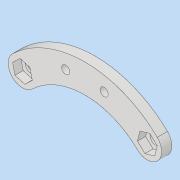
# Autodesk Inventor part: gearboxBearingHolderHexNutBacking
Saved by Autodesk Inventor 2017.3 (Build 213256000, 256)
## iProperties
Created: 2018-09-03
Part Number: gearboxBearingHolderHexNutBacking
Material: ABS Plastic
Document SubType Name: Modeling
Designer: Derek Wider
Density: 1.06 g/cm^3
Appearance: Smooth - White
Author: Derek Wider
Autodesk Inventor part; units mm, degrees
ref_plane "YZ Plane" through (0, 0, 0) normal (1, 0, 0) x (0, 1, 0)
ref_plane "XZ Plane" through (0, 0, 0) normal (0, 1, 0) x (-1, 0, 0)
ref_plane "XY Plane" through (0, 0, 0) normal (0, 0, 1) x (1, 0, 0)
sketch "Sketch1" plane through (0, 0, 0) normal (0, 0, 1) x (1, 0, 0)
  line L0 (-2.3083, -2.2118) -> (-3.0696, 0.8931)
  line L1 (-3.0696, 0.8931) -> (-0.7613, 3.1049)
  line L2 (-0.7613, 3.1049) -> (2.3083, 2.2118)
  line L3 (2.3083, 2.2118) -> (3.0696, -0.8931)
  line L4 (3.0696, -0.8931) -> (0.7613, -3.1049)
  line L5 (0.7613, -3.1049) -> (-2.3083, -2.2118)
  line L6 (41.9062, 0.8931) -> (41.1449, -2.2118)
  line L7 (41.1449, -2.2118) -> (38.0753, -3.1049)
  line L8 (38.0753, -3.1049) -> (35.767, -0.8931)
  line L9 (35.767, -0.8931) -> (36.5283, 2.2118)
  line L10 (36.5283, 2.2118) -> (39.5979, 3.1049)
  line L11 (39.5979, 3.1049) -> (41.9062, 0.8931)
  circle A0 centre (0, 0) radius 4.445
  circle A1 centre (38.8366, 0) radius 4.445
  arc A2 (41.9119, 3.2095) -> (-3.0753, 3.2095) centre (19.4183, -20.2654) ccw
  arc A3 (35.7613, -3.2095) -> (3.0753, -3.2095) centre (19.4183, -20.2654) ccw
  arc A4 (38.8366, 0) -> (0, 0) centre (19.4183, -20.2654) ccw construction
  line L12 (-1.9155, 1.999) -> (-3.0753, 3.2095) construction
  line L13 (40.7521, 1.999) -> (41.9119, 3.2095) construction
  circle A5 centre (13.4501, 7.1597) radius 1.27
  circle A6 centre (25.3865, 7.1597) radius 1.27
  dimension "d0" = 38.8366
  dimension "d1" = 5.5372
  dimension "d2" = 8.89
  dimension "d3" = 28.067
  dimension "d8" = 2.54
  dimension "d9" = 2.54
  dimension "d10" = 31.5
  dimension "d11" = 31.5
  constraints: 28 end point, 12 point on circle, 7 centre point, 5 coincident, 4 tangent, 2 line through centre, 2 midpoint, 2 perpendicular, 1 equal length, 1 equal radius, 1 horizontal alignment, 26 other
  measures "d0" distance of point (38.837, 0) point (0, 0)
  measures "d1" distance between parallel lines of L7 L10
  measures "d2" diameter of A0
  measures "d3" radius of A4
  measures "d8" diameter of A5
  measures "d9" diameter of A6
extrude "Extrusion1" add sketch "Sketch1" along normal blind 2.54
sketch "Sketch2" plane through (0, 0, 0) normal (0, 0, -1) x (-1, 0, 0)
  line L0 (0.7613, 3.1049) -> (3.0696, 0.8931) projected
  line L1 (3.0696, 0.8931) -> (2.3083, -2.2118) projected
  line L2 (2.3083, -2.2118) -> (-0.7613, -3.1049) projected
  line L3 (-0.7613, -3.1049) -> (-3.0696, -0.8931) projected
  line L4 (-3.0696, -0.8931) -> (-2.3083, 2.2118) projected
  line L5 (-2.3083, 2.2118) -> (0.7613, 3.1049) projected
  line L6 (-38.0753, -3.1049) -> (-41.1449, -2.2118) projected
  line L7 (-41.1449, -2.2118) -> (-41.9062, 0.8931) projected
  line L8 (-41.9062, 0.8931) -> (-39.5979, 3.1049) projected
  line L9 (-39.5979, 3.1049) -> (-36.5283, 2.2118) projected
  line L10 (-36.5283, 2.2118) -> (-35.767, -0.8931) projected
  line L11 (-35.767, -0.8931) -> (-38.0753, -3.1049) projected
  arc A0 (-41.9119, 3.2095) -> (-35.7613, -3.2095) centre (-38.8366, 0) ccw projected
  arc A1 (-3.0753, -3.2095) -> (-35.7613, -3.2095) centre (-19.4183, -20.2654) ccw projected
  arc A2 (-3.0753, -3.2095) -> (3.0753, 3.2095) centre (0, 0) ccw projected
  arc A3 (3.0753, 3.2095) -> (-41.9119, 3.2095) centre (-19.4183, -20.2654) ccw projected
  circle A4 centre (-25.3865, 7.1597) radius 1.27 projected
  circle A5 centre (-13.4501, 7.1597) radius 1.27 projected
  line L12 (0.7613, 3.1049) -> (3.0696, 0.8931) projected
  line L13 (3.0696, 0.8931) -> (2.3083, -2.2118) projected
  line L14 (2.3083, -2.2118) -> (-0.7613, -3.1049) projected
  line L15 (-0.7613, -3.1049) -> (-3.0696, -0.8931) projected
  line L16 (-3.0696, -0.8931) -> (-2.3083, 2.2118) projected
  line L17 (-2.3083, 2.2118) -> (0.7613, 3.1049) projected
  line L18 (-38.0753, -3.1049) -> (-41.1449, -2.2118) projected
  line L19 (-41.1449, -2.2118) -> (-41.9062, 0.8931) projected
  line L20 (-41.9062, 0.8931) -> (-39.5979, 3.1049) projected
  line L21 (-39.5979, 3.1049) -> (-36.5283, 2.2118) projected
  line L22 (-36.5283, 2.2118) -> (-35.767, -0.8931) projected
  line L23 (-35.767, -0.8931) -> (-38.0753, -3.1049) projected
  arc A6 (-41.9119, 3.2095) -> (-35.7613, -3.2095) centre (-38.8366, 0) ccw projected
  arc A7 (-3.0753, -3.2095) -> (-35.7613, -3.2095) centre (-19.4183, -20.2654) ccw projected
  arc A8 (-3.0753, -3.2095) -> (3.0753, 3.2095) centre (0, 0) ccw projected
  arc A9 (3.0753, 3.2095) -> (-41.9119, 3.2095) centre (-19.4183, -20.2654) ccw projected
  circle A10 centre (0, 0) radius 1.7145
  circle A11 centre (-38.8366, 0) radius 1.7145
  dimension "d12" = 3.429
  constraints: 2 centre point, 2 coincident, 1 equal radius
  measures "d12" diameter of A10
extrude "Extrusion2" add sketch "Sketch2" along normal blind 0.635 contours L0 L1 L2 L3 L4 L5 | L6 L7 L8 L9 L10 L11 | A3 A2 A1 A0
equation "\"d11\" = d10"
body "Solid1"
